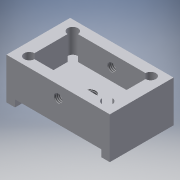
# Autodesk Inventor part: Küvettenklammer_20mm_version3
Saved by Autodesk Inventor 2016 (Build 200138000, 138)
## iProperties
Created: 2015-10-07
Part Number: Küvettenklammer_20mm_version3
Material: Allgemein
Document SubType Name: Modeling
Designer: voigt
Density: 1 g/cm^3
Appearance: PTFE
Author: voigt
Autodesk Inventor part; units mm, degrees
ref_plane "YZ Plane" through (0, 0, 0) normal (1, 0, 0) x (0, 1, 0)
ref_plane "XZ Plane" through (0, 0, 0) normal (0, 1, 0) x (-1, 0, 0)
ref_plane "XY Plane" through (0, 0, 0) normal (0, 0, 1) x (1, 0, 0)
sketch "Sketch1" plane through (0, 0, 0) normal (0, 0, 1) x (1, 0, 0)
  line L0 (0, 12.95) -> (0, -12.95) construction
  line L1 (-21, 0) -> (21, 0) construction
  line L2 (-15, 9.25) -> (15, 9.25)
  line L3 (15, 9.25) -> (15, -9.25)
  line L4 (15, -9.25) -> (-15, -9.25)
  line L5 (-15, -9.25) -> (-15, 9.25)
  point P0 (0, 0)
  dimension "d0" = 18.5
  dimension "d1" = 30
  constraints: 8 end point, 2 parallel, 1 horizontal, 1 perpendicular, 2 other
  measures "d0" distance of L4.end L2.start
  measures "d1" distance of L2.start L2.end
extrude "Extrusion1" add sketch "Sketch1" along normal blind 12
sketch "Sketch2" plane through (0, 0, 0) normal (0, 0, -1) x (-1, 0, 0)
  line L0 (-15, 9.25) -> (15, -9.25) construction
  line L1 (15, 9.25) -> (-15, -9.25) construction
  point P0 (0, 0)
  point P1 (0, 0)
  constraints: 4 end point, 1 coincident
hole "Hole1" at (0, 0, 0) direction (0, 0, 1) diameter 3.242 end through all thread size "M4x0.7" class "6H" standard "ISO Metric profile"
sketch "Sketch3" plane through (0, 0, 12) normal (0, 0, 1) x (1, 0, 0)
  line L0 (15, 9.25) -> (15, -9.25) projected
  line L1 (-15, 9.25) -> (15, 9.25) projected
  line L2 (-15, -9.25) -> (-15, 9.25) projected
  line L3 (15, -9.25) -> (-15, -9.25) projected
  line L4 (-15, 0) -> (15, 0) construction
  line L5 (0, 9.25) -> (0, -9.25) construction
  line L6 (-11.3, 6.3) -> (11.3, 6.3) construction
  line L7 (11.3, 6.3) -> (11.3, -6.3) construction
  line L8 (11.3, -6.3) -> (-11.3, -6.3) construction
  line L9 (-11.3, -6.3) -> (-11.3, 6.3) construction
  dimension "d11" = 12.6
  dimension "d12" = 22.6
  constraints: 12 end point, 4 coincident, 4 midpoint, 2 parallel, 1 horizontal, 1 perpendicular, 2 other
  measures "d11" distance of L6.end L7.end
  measures "d12" distance of L7.end L8.end
hole "Hole2" at (-11.3, 6.3, 12) at (11.3, 6.3, 12) at (11.3, -6.3, 12) at (-11.3, -6.3, 12) direction (0, 0, -1) diameter 3 depth 7
sketch "Sketch4" plane through (0, 0, 12) normal (0, 0, 1) x (1, 0, 0)
  circle A0 centre (11.3, -6.3) radius 1.5 projected
  circle A1 centre (-11.3, 6.3) radius 1.5 projected
  circle A2 centre (0, 0) radius 1.621 projected
  line L0 (-11.3, 6.3) -> (11.3, 6.3)
  line L1 (11.3, 6.3) -> (11.3, -6.3)
  line L2 (11.3, -6.3) -> (-11.3, -6.3)
  line L3 (-11.3, -6.3) -> (-11.3, 6.3)
  constraints: 8 end point, 2 parallel, 1 horizontal, 1 perpendicular
extrude "Extrusion2" cut sketch "Sketch4" against normal blind 7 contours L1 L2 A0 | A0 L2 L3 A1 L0 L1 | A1 L3 L0 picked at (10.3125, -6.1887) picked at (-10.4586, 5.7713)
sketch "Sketch5" plane through (-15, 9.25, 0) normal (0, 1, 0) x (1, 0, 0)
  line L0 (5.2, -12) -> (5.2, -5) construction
  line L1 (24.8, -12) -> (5.2, -12) construction
  line L2 (24.8, -5) -> (24.8, -12) construction
  line L3 (5.2, -5) -> (24.8, -5) construction
  line L4 (24.8, -8.5) -> (5.2, -8.5) construction
  point P0 (15, 0)
  point P1 (15, -8.5)
  dimension "d33" = 9.8
  constraints: 3 midpoint, 2 end point
  measures "d33" distance from line of L2 point (15, -8.5)
hole "Hole3" at (0, 9.25, 8.5) direction (0, -1, 0) diameter 2.459 end through all thread size "M3x0.5" class "6H" standard "ANSI Metric M Profile"
sketch "Sketch6" plane through (-15, 9.25, 0) normal (0, 1, 0) x (1, 0, 0)
  line L0 (0, 0) -> (30, 0) projected
  line L1 (15, 2.4) -> (15, -14.4) construction
  line L2 (2.5, 0) -> (27.5, 0)
  line L3 (27.5, 0) -> (27.5, -2)
  line L4 (27.5, -2) -> (2.5, -2)
  line L5 (2.5, -2) -> (2.5, 0)
  point P0 (15, 0)
  dimension "d29" = 25
  dimension "d30" = 2
  constraints: 8 end point, 2 parallel, 1 horizontal, 1 perpendicular, 1 point on line, 1 other
  measures "d29" distance of L3.end L4.end
  measures "d30" distance of L2.end L3.end
extrude "Extrusion3" cut sketch "Sketch6" against normal up to next
body "Solid1"
